Autodesk Fusion 360 part; units mm, degrees
(part 3 of 4)
sketch "Skizze42" plane through (0, 47, 0) normal (0, 1, 0) x (-1, 0, 0)
  line L0 (22.3, -10.5) -> (30, -10.5)
  line L1 (30, -10.5) -> (30, -18.5)
  line L2 (30, -18.5) -> (22.3, -18.5)
  line L3 (22.3, -18.5) -> (22.3, -10.5)
  line L4 (-37.3325, -7.5) -> (-48.5, -7.5)
  arc A0 (-48.5, -4.5) -> (-48.5, -7.5) centre (-48.5, -6) ccw
  line L5 (-48.5, -4.5) -> (-37.3325, -4.5)
  arc A1 (-37.3325, -7.5) -> (-37.3325, -4.5) centre (-37.3325, -6) ccw
  line L6 (-12.5, -6.3514) -> (-20.5, -6.3514)
  arc A2 (-20.5, -4.3514) -> (-20.5, -6.3514) centre (-20.5, -5.3514) ccw
  line L7 (-20.5, -4.3514) -> (-12.5, -4.3514)
  arc A3 (-12.5, -6.3514) -> (-12.5, -4.3514) centre (-12.5, -5.3514) ccw
  line L8 (-12.5, -24.0657) -> (-20.5, -24.0657)
  arc A4 (-20.5, -22.0657) -> (-20.5, -24.0657) centre (-20.5, -23.0657) ccw
  line L9 (-20.5, -22.0657) -> (-12.5, -22.0657)
  arc A5 (-12.5, -24.0657) -> (-12.5, -22.0657) centre (-12.5, -23.0657) ccw
  arc A6 (34, -4.5) -> (34, -7.5) centre (34, -6) ccw
  line L10 (34, -4.5) -> (45, -4.5)
  arc A7 (45, -7.5) -> (45, -4.5) centre (45, -6) ccw
  line L11 (45, -7.5) -> (34, -7.5)
  line L12 (34, 1.5) -> (45, 1.5)
  arc A8 (45, -1.5) -> (45, 1.5) centre (45, 0) ccw
  line L13 (45, -1.5) -> (34, -1.5)
  arc A9 (34, 1.5) -> (34, -1.5) centre (34, 0) ccw
  line L14 (-12.5, -19.6371) -> (-20.5, -19.6371)
  arc A10 (-20.5, -17.6371) -> (-20.5, -19.6371) centre (-20.5, -18.6371) ccw
  line L15 (-20.5, -17.6371) -> (-12.5, -17.6371)
  arc A11 (-12.5, -19.6371) -> (-12.5, -17.6371) centre (-12.5, -18.6371) ccw
  arc A12 (-20.8852, 0) -> (-20.5, -1.9228) centre (-20.5, -0.9228) ccw
  line L16 (-20.8852, 0) -> (-12.1148, 0)
  arc A13 (-12.5, -1.9228) -> (-12.1148, 0) centre (-12.5, -0.9228) ccw
  line L17 (-12.5, -1.9228) -> (-20.5, -1.9228)
  line L18 (-37.3325, -1.5) -> (-48.5, -1.5)
  arc A14 (-48.5, 1.5) -> (-48.5, -1.5) centre (-48.5, 0) ccw
  line L19 (-48.5, 1.5) -> (-37.3325, 1.5)
  arc A15 (-37.3325, -1.5) -> (-37.3325, 1.5) centre (-37.3325, 0) ccw
  line L20 (-20.5, 8.9343) -> (-12.5, 8.9343)
  arc A16 (-12.5, 6.9343) -> (-12.5, 8.9343) centre (-12.5, 7.9343) ccw
  line L21 (-12.5, 6.9343) -> (-20.5, 6.9343)
  arc A17 (-20.5, 8.9343) -> (-20.5, 6.9343) centre (-20.5, 7.9343) ccw
  line L22 (-12.5, -10.78) -> (-20.5, -10.78)
  arc A18 (-20.5, -8.78) -> (-20.5, -10.78) centre (-20.5, -9.78) ccw
  line L23 (-20.5, -8.78) -> (-12.5, -8.78)
  arc A19 (-12.5, -10.78) -> (-12.5, -8.78) centre (-12.5, -9.78) ccw
  arc A20 (34, 13.5) -> (34, 10.5) centre (34, 12) ccw
  line L24 (34, 13.5) -> (45, 13.5)
  arc A21 (45, 10.5) -> (45, 13.5) centre (45, 12) ccw
  line L25 (45, 10.5) -> (34, 10.5)
  arc A22 (34, -10.5) -> (34, -13.5) centre (34, -12) ccw
  line L26 (34, -10.5) -> (45, -10.5)
  arc A23 (45, -13.5) -> (45, -10.5) centre (45, -12) ccw
  line L27 (45, -13.5) -> (34, -13.5)
  arc A24 (34, 7.5) -> (34, 4.5) centre (34, 6) ccw
  line L28 (34, 7.5) -> (45, 7.5)
  arc A25 (45, 4.5) -> (45, 7.5) centre (45, 6) ccw
  line L29 (45, 4.5) -> (34, 4.5)
  line L30 (-12.5, -15.2086) -> (-20.5, -15.2086)
  arc A26 (-20.5, -13.2086) -> (-20.5, -15.2086) centre (-20.5, -14.2086) ccw
  line L31 (-20.5, -13.2086) -> (-12.5, -13.2086)
  arc A27 (-12.5, -15.2086) -> (-12.5, -13.2086) centre (-12.5, -14.2086) ccw
  line L32 (-12.5, 2.5057) -> (-20.5, 2.5057)
  arc A28 (-20.5, 4.5057) -> (-20.5, 2.5057) centre (-20.5, 3.5057) ccw
  line L33 (-20.5, 4.5057) -> (-12.5, 4.5057)
  arc A29 (-12.5, 2.5057) -> (-12.5, 4.5057) centre (-12.5, 3.5057) ccw
  line L34 (-37.3325, 4.5) -> (-48.5, 4.5)
  arc A30 (-48.5, 7.5) -> (-48.5, 4.5) centre (-48.5, 6) ccw
  line L35 (-48.5, 7.5) -> (-37.3325, 7.5)
  arc A31 (-37.3325, 4.5) -> (-37.3325, 7.5) centre (-37.3325, 6) ccw
  line L36 (21.5, -1.5) -> (21.5, -23.5)
  line L37 (21.5, -23.5) -> (-5.5, -23.5)
  line L38 (-5.5, -23.5) -> (-5.5, -1.5)
  line L39 (-5.5, -1.5) -> (21.5, -1.5)
  circle A32 centre (-36, 14.5) radius 1.9
  circle A33 centre (36, 25) radius 1.9
  circle A34 centre (36, -25) radius 1.9
  circle A35 centre (-36, -14.5) radius 1.9
  line L40 (-12, 21.5) -> (-12, 11.5)
  line L41 (-12, 11.5) -> (-21, 11.5)
  line L42 (-21, 11.5) -> (-21, 21.5)
  line L43 (-21, 21.5) -> (-22.5, 21.5)
  line L44 (-22.5, 21.5) -> (-22.5, 27.5)
  line L45 (-22.5, 27.5) -> (-32.5, 27.5)
  line L46 (-32.5, 27.5) -> (-32.5, 19)
  arc A36 (-33.5, 18) -> (-32.5, 19) centre (-33.5, 19) ccw
  line L47 (-33.5, 18) -> (-40.5, 18)
  line L48 (-40.5, 18) -> (-40.5, 11)
  line L49 (-40.5, 11) -> (-56.5, 11)
  line L50 (-56.5, 11) -> (-56.5, -11)
  line L51 (-56.5, -11) -> (-40.5, -11)
  line L52 (-40.5, -11) -> (-40.5, -18)
  line L53 (-40.5, -18) -> (-33.5, -18)
  arc A37 (-32.5, -19) -> (-33.5, -18) centre (-33.5, -19) ccw
  line L54 (-32.5, -19) -> (-32.5, -27.5)
  line L55 (-32.5, -27.5) -> (32.5, -27.5)
  line L56 (32.5, -27.5) -> (33.8276, -28.3587)
  arc A38 (33.8276, -28.3587) -> (39.5022, -26.9326) centre (36, -25) ccw
  line L57 (39.5022, -26.9326) -> (42.5, -21.5)
  line L58 (42.5, -21.5) -> (57.5, -6.5)
  line L59 (57.5, -6.5) -> (57.5, 6.5)
  line L60 (57.5, 6.5) -> (42.5, 21.5)
  line L61 (42.5, 21.5) -> (39.5022, 26.9326)
  arc A39 (39.5022, 26.9326) -> (33.8276, 28.3587) centre (36, 25) ccw
  line L62 (33.8276, 28.3587) -> (32.5, 27.5)
  line L63 (32.5, 27.5) -> (-10.5, 27.5)
  line L64 (-10.5, 27.5) -> (-10.5, 21.5)
  line L65 (-10.5, 21.5) -> (-12, 21.5)
  circle A40 centre (3.5, 16) radius 6.5
  line L66 (51.5218, -5) -> (57.5, -5)
  line L67 (57.5, -5) -> (57.5, -6.5)
  line L68 (57.5, -6.5) -> (42.5, -21.5)
  line L69 (32.5, -27.5) -> (-32.5, -27.5)
  line L70 (-32.5, -27.5) -> (-32.5, -19)
  line L71 (-32.5, -19) -> (-31, -19)
  line L72 (-31, -19) -> (-31, -26)
  line L73 (-31, -26) -> (-23, -26)
  line L74 (-23, -26) -> (23, -26)
  line L75 (23, -26) -> (31, -26)
  line L76 (31, -26) -> (31, -20)
  line L77 (31, -20) -> (41.8787, -20)
  line L78 (41.8787, -20) -> (51.5218, -10.3569)
  line L79 (51.5218, -10.3569) -> (51.5218, -5)
  circle A41 centre (36, -25) radius 1.9
  line L80 (57.5, 5) -> (51.5218, 5)
  line L81 (51.5218, 5) -> (51.5218, 10.3569)
  line L82 (51.5218, 10.3569) -> (41.8787, 20)
  line L83 (41.8787, 20) -> (31, 20)
  line L84 (31, 20) -> (31, 26)
  line L85 (31, 26) -> (-31, 26)
  line L86 (-31, 26) -> (-31, 19)
  line L87 (-31, 19) -> (-32.5, 19)
  line L88 (-32.5, 19) -> (-32.5, 27.5)
  line L89 (-32.5, 27.5) -> (32.5, 27.5)
  line L90 (42.5, 21.5) -> (57.5, 6.5)
  line L91 (57.5, 6.5) -> (57.5, 5)
  circle A42 centre (36, 25) radius 1.9
  line L92 (-51.5, 5) -> (-56.5, 5)
  line L93 (-56.5, 5) -> (-56.5, 11)
  line L94 (-56.5, 11) -> (-40.5, 11)
  line L95 (-38.5, 18) -> (-33.5, 18)
  arc A43 (-33.5, 18) -> (-32.5, 19) centre (-33.5, 19) ccw
  line L96 (-32.5, 19) -> (-31, 19)
  line L97 (-31, 19) -> (-31, 9.5)
  line L98 (-31, 9.5) -> (-51.5, 9.5)
  line L99 (-51.5, 9.5) -> (-51.5, 5)
  circle A44 centre (-36, 14.5) radius 1.9
  line L100 (-56.5, -5) -> (-51.5, -5)
  line L101 (-51.5, -5) -> (-51.5, -9.5)
  line L102 (-51.5, -9.5) -> (-31, -9.5)
  line L103 (-31, -9.5) -> (-31, -19)
  line L104 (-31, -19) -> (-32.5, -19)
  arc A45 (-32.5, -19) -> (-33.5, -18) centre (-33.5, -19) ccw
  line L105 (-33.5, -18) -> (-38.5, -18)
  line L106 (-40.5, -11) -> (-56.5, -11)
  line L107 (-56.5, -11) -> (-56.5, -5)
  circle A46 centre (-36, -14.5) radius 1.9
  circle A47 centre (36, 25) radius 4
  circle A48 centre (-36, 14.5) radius 3.5
  circle A49 centre (-36, -14.5) radius 3.5
  line L108 (-32.5, 19) -> (-32.5, 14.5)
  line L109 (-40.5, 11) -> (-36, 11)
  line L110 (-40.5, -11) -> (-36, -11)
  line L111 (-32.5, -19) -> (-32.5, -14.5)
  line L112 (32, 25) -> (32, 27.5)
  line L113 (36, 21) -> (43, 21)
  line L114 (-1.75, 0) -> (-22.5, 0)
  line L115 (36, -21) -> (43, -21)
  circle A50 centre (36, -25) radius 4
  line L116 (32, -25) -> (32, -27.5)
  line L117 (42.5, -21.5) -> (38.922, -26.9266)
  arc A51 (34.8649, -28.3108) -> (38.922, -26.9266) centre (36, -25) ccw
  line L118 (34.8649, -28.3108) -> (32.5, -27.5)
  line L119 (32.5, 27.5) -> (34.8649, 28.3108)
  arc A52 (38.922, 26.9266) -> (34.8649, 28.3108) centre (36, 25) ccw
  line L120 (38.922, 26.9266) -> (42.5, 21.5)
  arc A53 (-40.5, 11) -> (-39.5, 12) centre (-40.5, 12) ccw
  line L121 (-39.5, 12) -> (-39.5, 17)
  arc A54 (-38.5, 18) -> (-39.5, 17) centre (-38.5, 17) ccw
  arc A55 (-39.5, -17) -> (-38.5, -18) centre (-38.5, -17) ccw
  line L122 (-39.5, -17) -> (-39.5, -12)
  arc A56 (-39.5, -12) -> (-40.5, -11) centre (-40.5, -12) ccw
  dimension "d212" = 7
  dimension "d213" = 7
  measures "d212" diameter of A48
  measures "d213" diameter of A49
extrude "Extrusion42" cut sketch "Skizze42" against normal blind 13.5 contours L63 L89 A47 L112 L119 | L62 A47 L119 | A47 L119 A52 L120 | A39 A47 L119 A52 L120 | L60 L90 A47 L113 L120 | A36 L47 L95 A43 A48 L108 | L61 A47 L120 | A48 | L47 L95 A48 L121 A54 | A48 L109 A53 L121 | L47 L48 A53 L121 A54 | L58 L68 L115 A50 L117 | L57 A50 L117 | A50 L117 A51 L118 | L52 L53 A55 L122 A56 | A49 L110 L122 A56 | A38 A50 L117 A51 L118 | L55 L69 A50 L116 L118 | A49 | L56 A50 L118 | L53 L105 A49 A55 L122 | L53 A37 A45 L105 A49 L111 bodies 2
fillet "Abrundung2" radius 1 8 edges at (40.5, 10.75, 18) (40.5, 10.75, 11) (40.5, 10.75, -11) (40.5, 10.75, -18) (40.5, 29, 18) (40.5, 29, 11) (40.5, 29, -11) (40.5, 29, -18) on bodies 1 2
sketch "Skizze43" plane through (-32, 0, 32) normal (-0.707107, 0, 0.707107) x (0.707107, 0, 0.707107)
  line L0 (-15.5563, 33.5) -> (-15.5563, 47)
  line L1 (-15.5563, 47) -> (-36.0624, 47)
  line L2 (-36.0624, 47) -> (-36.0624, 16)
  line L3 (-36.0624, 16) -> (-14.8492, 16)
  line L4 (-14.8492, 19) -> (-14.8492, 33.5)
  line L5 (-14.8492, 33.5) -> (-15.5563, 33.5)
  circle A0 centre (-21.4706, 18) radius 2
  line L6 (-29.108, 16) -> (-29.108, 45)
  line L7 (-29.108, 45) -> (-15.4706, 45)
  line L8 (-15.4706, 45) -> (-15.4706, 16)
  line L9 (-15.4706, 16) -> (-29.108, 16)
  line L10 (-14.8492, 16) -> (-36.0624, 16)
  line L11 (-23.0518, 16) -> (-20.1969, 16)
  line L12 (-23.4706, 16) -> (-19.4706, 16)
  line L13 (-19.4706, 16) -> (-19.4706, 18)
  line L14 (-19.4706, 18) -> (-23.4706, 18)
  line L15 (-23.4706, 18) -> (-23.4706, 16)
  line L16 (-14.8492, 16) -> (-14.8492, 19)
  dimension "d217" = 4
  dimension "d223" = 6
  measures "d217" diameter of A0
  measures "d223" distance of L8
extrude "Extrusion43" cut sketch "Skizze43" against normal blind 2 contours L3 A0 L9 L10 L11 L12 L13 | L3 A0 L9 L10 L11 L12 L15 | A0 L14 | A0 L14 bodies 2
sketch "Sketch44" plane through (0, 47, 0) normal (0, 1, 0) x (-1, 0, 0)
  circle A0 centre (3.5, 16) radius 6.5
  line L0 (21.5, -1.5) -> (21.5, -23.5)
  line L1 (21.5, -23.5) -> (-5.5, -23.5)
  line L2 (-5.5, -23.5) -> (-5.5, -1.5)
  line L3 (-5.5, -1.5) -> (21.5, -1.5)
  line L4 (-37.3325, 4.5) -> (-48.5, 4.5)
  arc A1 (-48.5, 7.5) -> (-48.5, 4.5) centre (-48.5, 6) ccw
  line L5 (-48.5, 7.5) -> (-37.3325, 7.5)
  arc A2 (-37.3325, 4.5) -> (-37.3325, 7.5) centre (-37.3325, 6) ccw
  line L6 (-12.5, 2.5057) -> (-20.5, 2.5057)
  arc A3 (-20.5, 4.5057) -> (-20.5, 2.5057) centre (-20.5, 3.5057) ccw
  line L7 (-20.5, 4.5057) -> (-12.5, 4.5057)
  arc A4 (-12.5, 2.5057) -> (-12.5, 4.5057) centre (-12.5, 3.5057) ccw
  line L8 (-12.5, -15.2086) -> (-20.5, -15.2086)
  arc A5 (-20.5, -13.2086) -> (-20.5, -15.2086) centre (-20.5, -14.2086) ccw
  line L9 (-20.5, -13.2086) -> (-12.5, -13.2086)
  arc A6 (-12.5, -15.2086) -> (-12.5, -13.2086) centre (-12.5, -14.2086) ccw
  arc A7 (34, 7.5) -> (34, 4.5) centre (34, 6) ccw
  line L10 (34, 7.5) -> (45, 7.5)
  arc A8 (45, 4.5) -> (45, 7.5) centre (45, 6) ccw
  line L11 (45, 4.5) -> (34, 4.5)
  arc A9 (34, -10.5) -> (34, -13.5) centre (34, -12) ccw
  line L12 (34, -10.5) -> (45, -10.5)
  arc A10 (45, -13.5) -> (45, -10.5) centre (45, -12) ccw
  line L13 (45, -13.5) -> (34, -13.5)
  arc A11 (34, 13.5) -> (34, 10.5) centre (34, 12) ccw
  line L14 (34, 13.5) -> (45, 13.5)
  arc A12 (45, 10.5) -> (45, 13.5) centre (45, 12) ccw
  line L15 (45, 10.5) -> (34, 10.5)
  line L16 (-12.5, -10.78) -> (-20.5, -10.78)
  arc A13 (-20.5, -8.78) -> (-20.5, -10.78) centre (-20.5, -9.78) ccw
  line L17 (-20.5, -8.78) -> (-12.5, -8.78)
  arc A14 (-12.5, -10.78) -> (-12.5, -8.78) centre (-12.5, -9.78) ccw
  line L18 (-20.5, 8.9343) -> (-12.5, 8.9343)
  arc A15 (-12.5, 6.9343) -> (-12.5, 8.9343) centre (-12.5, 7.9343) ccw
  line L19 (-12.5, 6.9343) -> (-20.5, 6.9343)
  arc A16 (-20.5, 8.9343) -> (-20.5, 6.9343) centre (-20.5, 7.9343) ccw
  line L20 (-37.3325, -1.5) -> (-48.5, -1.5)
  arc A17 (-48.5, 1.5) -> (-48.5, -1.5) centre (-48.5, 0) ccw
  line L21 (-48.5, 1.5) -> (-37.3325, 1.5)
  arc A18 (-37.3325, -1.5) -> (-37.3325, 1.5) centre (-37.3325, 0) ccw
  arc A19 (-20.8852, 0) -> (-20.5, -1.9228) centre (-20.5, -0.9228) ccw
  line L22 (-20.8852, 0) -> (-12.1148, 0)
  arc A20 (-12.5, -1.9228) -> (-12.1148, 0) centre (-12.5, -0.9228) ccw
  line L23 (-12.5, -1.9228) -> (-20.5, -1.9228)
  line L24 (-12.5, -19.6371) -> (-20.5, -19.6371)
  arc A21 (-20.5, -17.6371) -> (-20.5, -19.6371) centre (-20.5, -18.6371) ccw
  line L25 (-20.5, -17.6371) -> (-12.5, -17.6371)
  arc A22 (-12.5, -19.6371) -> (-12.5, -17.6371) centre (-12.5, -18.6371) ccw
  line L26 (34, 1.5) -> (45, 1.5)
  arc A23 (45, -1.5) -> (45, 1.5) centre (45, 0) ccw
  line L27 (45, -1.5) -> (34, -1.5)
  arc A24 (34, 1.5) -> (34, -1.5) centre (34, 0) ccw
  arc A25 (34, -4.5) -> (34, -7.5) centre (34, -6) ccw
  line L28 (34, -4.5) -> (45, -4.5)
  arc A26 (45, -7.5) -> (45, -4.5) centre (45, -6) ccw
  line L29 (45, -7.5) -> (34, -7.5)
  line L30 (-12.5, -24.0657) -> (-20.5, -24.0657)
  arc A27 (-20.5, -22.0657) -> (-20.5, -24.0657) centre (-20.5, -23.0657) ccw
  line L31 (-20.5, -22.0657) -> (-12.5, -22.0657)
  arc A28 (-12.5, -24.0657) -> (-12.5, -22.0657) centre (-12.5, -23.0657) ccw
  line L32 (-12.5, -6.3514) -> (-20.5, -6.3514)
  arc A29 (-20.5, -4.3514) -> (-20.5, -6.3514) centre (-20.5, -5.3514) ccw
  line L33 (-20.5, -4.3514) -> (-12.5, -4.3514)
  arc A30 (-12.5, -6.3514) -> (-12.5, -4.3514) centre (-12.5, -5.3514) ccw
  line L34 (-37.3325, -7.5) -> (-48.5, -7.5)
  arc A31 (-48.5, -4.5) -> (-48.5, -7.5) centre (-48.5, -6) ccw
  line L35 (-48.5, -4.5) -> (-37.3325, -4.5)
  arc A32 (-37.3325, -7.5) -> (-37.3325, -4.5) centre (-37.3325, -6) ccw
  line L36 (22.3, -10.5) -> (30, -10.5)
  line L37 (30, -10.5) -> (30, -18.5)
  line L38 (30, -18.5) -> (22.3, -18.5)
  line L39 (22.3, -18.5) -> (22.3, -10.5)
  line L40 (-32.5, 27.5) -> (-32.5, 14.5)
  arc A33 (-36, 11) -> (-32.5, 14.5) centre (-36, 14.5) ccw
  line L41 (-36, 11) -> (-56.5, 11)
  line L42 (-56.5, 11) -> (-56.5, -11)
  line L43 (-56.5, -11) -> (-36, -11)
  arc A34 (-32.5, -14.5) -> (-36, -11) centre (-36, -14.5) ccw
  line L44 (-32.5, -14.5) -> (-32.5, -27.5)
  line L45 (-32.5, -27.5) -> (32, -27.5)
  line L46 (32, -27.5) -> (32, -25)
  arc A35 (36, -21) -> (32, -25) centre (36, -25) ccw
  line L47 (36, -21) -> (43, -21)
  line L48 (43, -21) -> (57.5, -6.5)
  line L49 (57.5, -6.5) -> (57.5, 6.5)
  line L50 (57.5, 6.5) -> (43, 21)
  line L51 (43, 21) -> (36, 21)
  arc A36 (32, 25) -> (36, 21) centre (36, 25) ccw
  line L52 (32, 25) -> (32, 27.5)
  line L53 (32, 27.5) -> (-10.5, 27.5)
  line L54 (-10.5, 27.5) -> (-10.5, 21.5)
  line L55 (-10.5, 21.5) -> (-12, 21.5)
  line L56 (-12, 21.5) -> (-12, 11.5)
  line L57 (-12, 11.5) -> (-21, 11.5)
  line L58 (-21, 11.5) -> (-21, 21.5)
  line L59 (-21, 21.5) -> (-22.5, 21.5)
  line L60 (-22.5, 21.5) -> (-22.5, 27.5)
  line L61 (-22.5, 27.5) -> (-32.5, 27.5)
  line L62 (-12.5, -4.3514) -> (-20.5, -4.3514)
  line L63 (-20.5, -4.3514) -> (-20.5, -7.58)
  line L64 (-20.5, -7.58) -> (-12.5, -7.58)
  line L65 (-12.5, -7.58) -> (-12.5, -4.3514)
  dimension "d220" = 1.2
  measures "d220" distance of L17 L64
extrude "Extrude44" cut sketch "Sketch44" against normal blind 2 contours L32 L63 L64 L65 bodies 2
sketch "Skizze46" plane through (0, 0, -27.5) normal (0, 0, -1) x (-1, 0, 0)
  line L0 (-32.5, 0) -> (32.5, 0)
  line L1 (32.5, 0) -> (32.5, 16)
  line L2 (32.5, 16) -> (-32.5, 16)
  line L3 (-32.5, 16) -> (-32.5, 0)
  line L4 (-20, 2) -> (20, 2)
  line L5 (20, 2) -> (20, 42)
  line L6 (20, 42) -> (-20, 42)
  line L7 (-20, 42) -> (-20, 2)
  circle A0 centre (0, 22) radius 19
  circle A1 centre (-16, 38) radius 1.75
  circle A2 centre (-16, 6) radius 1.75
  line L8 (0, 1.75) -> (0, 22.5)
  circle A3 centre (16, 38) radius 1.75
  circle A4 centre (16, 6) radius 1.75
  circle A5 centre (0, 22) radius 2
  line L9 (0, 22) -> (-16, 6)
  line L10 (-16, 6) -> (-16.7071, 6.7071)
  line L11 (-16.7071, 6.7071) -> (-0.7071, 22.7071)
  line L12 (-0.7071, 22.7071) -> (0, 22)
  line L13 (0, 22) -> (-16, 6)
  line L14 (-16, 6) -> (-15.2929, 5.2929)
  line L15 (-15.2929, 5.2929) -> (0.7071, 21.2929)
  line L16 (0.7071, 21.2929) -> (0, 22)
  line L17 (15.2929, 5.2929) -> (-0.7071, 21.2929)
  line L18 (16.7071, 6.7071) -> (0.7071, 22.7071)
  line L19 (16.7071, 37.2929) -> (0.7071, 21.2929)
  line L20 (15.2929, 38.7071) -> (-0.7071, 22.7071)
  line L21 (-15.2929, 38.7071) -> (0.7071, 22.7071)
  line L22 (-16.7071, 37.2929) -> (-0.7071, 21.2929)
  dimension "d224" = 40
  dimension "d225" = 40
  dimension "d226" = 12.5
  dimension "d227" = 38
  dimension "d228" = 3.5
  dimension "d229" = 20
  dimension "d230" = 20
  dimension "d231" = 4
  dimension "d232" = 4
  dimension "d233" = 3.5
  dimension "d234" = 4
  dimension "d235" = 4
  dimension "d236" = 4
  dimension "d237" = 1
  dimension "d238" = 1
  dimension "d240" = 360
  dimension "d241" = 2
  measures "d225" distance of origin
  measures "d226" distance of L3 L7
  measures "d227" diameter of A0
  measures "d228" diameter of A1
  measures "d229" distance of L7 origin
  measures "d230" distance of L4 origin
  measures "d232" distance of L7
  measures "d233" diameter of A2
  measures "d234" distance of L4
  measures "d235" distance of L7
  measures "d236" diameter of A5
  measures "d241" distance of L0 L4
extrude "Extrusion45" cut sketch "Skizze46" against normal blind 2 contours L2 A0 A5 L11 L22 | L2 A0 L11 | L2 A0 L18 | L2 A0 A5 L18 L19 | A0 A5 L20 L21 | A1 | A2 L10 L11 L14 L15 | A2 L9 L10 L11 L13 | L2 A0 L8 L17 | L2 A0 L8 L15 | L2 L8 A5 L17 | L2 L8 A5 L15 | A2 L9 L13 L14 L15 | A3 bodies 1 2
sketch "Skizze53" plane through (0, 0, -27.5) normal (0, 0, -1) x (-1, 0, 0)
  line L0 (4.5858, 16) -> (12.7093, 7.8765)
  arc A0 (-12.7093, 7.8765) -> (12.7093, 7.8765) centre (0, 22) ccw
  line L1 (-12.7093, 7.8765) -> (-4.5858, 16)
  line L2 (-4.5858, 16) -> (-7.4142, 16)
  line L3 (-7.4142, 16) -> (-14.1235, 9.2907)
  arc A1 (-18.0278, 16) -> (-14.1235, 9.2907) centre (0, 22) ccw
  line L4 (-18.0278, 16) -> (-32.5, 16)
  line L5 (-32.5, 16) -> (-32.5, 0)
  line L6 (-32.5, 0) -> (32.5, 0)
  line L7 (32.5, 0) -> (32.5, 16)
  line L8 (32.5, 16) -> (18.0278, 16)
  arc A2 (14.1235, 9.2907) -> (18.0278, 16) centre (0, 22) ccw
  line L9 (14.1235, 9.2907) -> (7.4142, 16)
  line L10 (7.4142, 16) -> (4.5858, 16)
  circle A3 centre (-16, 6) radius 1.75
  line L11 (-20, 2) -> (20, 2)
  line L12 (20, 2) -> (20, 42)
  line L13 (20, 42) -> (-20, 42)
  line L14 (-20, 42) -> (-20, 2)
  line L15 (0.5176, 20.0681) -> (4.5858, 16)
  line L16 (4.5858, 16) -> (7.4142, 16)
  line L17 (7.4142, 16) -> (1.9319, 21.4824)
  arc A4 (1.9319, 21.4824) -> (1.9319, 22.5176) centre (0, 22) ccw
  line L18 (1.9319, 22.5176) -> (14.1235, 34.7093)
  arc A5 (18.0278, 16) -> (14.1235, 34.7093) centre (0, 22) ccw
  line L19 (32.5, 19) -> (32.5, 33.5)
  line L20 (32.5, 33.5) -> (32, 33.5)
  line L21 (32, 33.5) -> (32, 47)
  line L22 (32, 47) -> (-32.5, 47)
  line L23 (-32.5, 47) -> (-32.5, 16)
  line L24 (-32.5, 16) -> (-18.0278, 16)
  arc A6 (-14.1235, 34.7093) -> (-18.0278, 16) centre (0, 22) ccw
  line L25 (-14.1235, 34.7093) -> (-1.9319, 22.5176)
  arc A7 (-1.9319, 22.5176) -> (-1.9319, 21.4824) centre (0, 22) ccw
  line L26 (-1.9319, 21.4824) -> (-7.4142, 16)
  line L27 (-7.4142, 16) -> (-4.5858, 16)
  line L28 (-4.5858, 16) -> (-0.5176, 20.0681)
  arc A8 (-0.5176, 20.0681) -> (0.5176, 20.0681) centre (0, 22) ccw
  circle A9 centre (-16, 38) radius 1.75
  circle A10 centre (16, 38) radius 1.75
  arc A11 (12.7093, 36.1235) -> (-12.7093, 36.1235) centre (0, 22) ccw
  line L29 (12.7093, 36.1235) -> (0.5176, 23.9319)
  arc A12 (0.5176, 23.9319) -> (-0.5176, 23.9319) centre (0, 22) ccw
  line L30 (-0.5176, 23.9319) -> (-12.7093, 36.1235)
  line L31 (-20, 42) -> (-13, 42)
  line L32 (-13, 42) -> (-13, 44)
  line L33 (-13, 44) -> (-20, 44)
  line L34 (-20, 44) -> (-20, 42)
  line L35 (-20, 44) -> (-22, 44)
  line L36 (-22, 44) -> (-22, 35.2606)
  line L37 (-22, 35.2606) -> (-20, 35.2606)
  line L38 (-20, 35.2606) -> (-20, 44)
  line L39 (20, 42) -> (13, 42)
  line L40 (13, 42) -> (13, 44)
  line L41 (13, 44) -> (20, 44)
  line L42 (20, 44) -> (20, 42)
  line L43 (20, 44) -> (22, 44)
  line L44 (22, 44) -> (22, 35)
  line L45 (22, 35) -> (20, 35)
  line L46 (20, 35) -> (20, 44)
  line L47 (-20, 2) -> (-13, 2)
  line L48 (-13, 2) -> (-13, 0)
  line L49 (-13, 0) -> (-20, 0)
  line L50 (-20, 0) -> (-20, 2)
  line L51 (-20, 0) -> (-22, 0)
  line L52 (-22, 0) -> (-22, 9)
  line L53 (-22, 9) -> (-20, 9)
  line L54 (-20, 9) -> (-20, 0)
  line L55 (20, 2) -> (13, 2)
  line L56 (13, 2) -> (13, 0)
  line L57 (13, 0) -> (20, 0)
  line L58 (20, 0) -> (20, 2)
  line L59 (20, 0) -> (22, 0)
  line L60 (22, 0) -> (22, 9)
  line L61 (22, 9) -> (20, 9)
  line L62 (20, 9) -> (20, 0)
  line L63 (18.0278, 16) -> (32.5, 16)
  line L64 (32.5, 16) -> (32.5, 19)
  dimension "d269" = 40
  dimension "d270" = 40
  dimension "d271" = 12.5
  dimension "d272" = 2
  dimension "d273" = 7
  dimension "d274" = 8.7394
  dimension "d275" = 2
  dimension "d276" = 7
  dimension "d277" = 9
  dimension "d278" = 2
  dimension "d279" = 7
  dimension "d280" = 2
  dimension "d281" = 9
  dimension "d282" = 7
  dimension "d283" = 9
  dimension "d284" = 2
  measures "d269" distance of origin
  measures "d271" distance of L5 L14
  measures "d272" distance of L6 L11
  measures "d273" distance of origin
  measures "d276" distance of origin
  measures "d281" distance of origin
  measures "d283" distance of origin
extrude "Extrusion54" add sketch "Skizze53" along normal blind 10.6 contours L6 L12 L58 L59 L60 L61 L62 | L12 L42 L43 L44 L45 L46 | L6 L11 L55 L56 L57 L58 L62 | L13 L39 L40 L41 L42 L46 | L14 L34 L35 L36 L37 L38 | L6 L14 L50 L51 L52 L53 L54 | L6 L11 L47 L48 L49 L50 L54 | L13 L31 L32 L33 L34 L38 bodies 1 2
sketch "Skizze54" plane through (0, 0, -38.1) normal (0, 0, -1) x (-1, 0, 0)
  line L0 (-20, 35.2606) -> (-20, 42)
  line L1 (-20, 42) -> (-13, 42)
  line L2 (-13, 42) -> (-13, 44)
  line L3 (-13, 44) -> (-22, 44)
  line L4 (-22, 44) -> (-22, 35.2606)
  line L5 (-22, 35.2606) -> (-20, 35.2606)
  line L6 (-13, 42) -> (-20, 35.2606)
  line L7 (20, 35) -> (22, 35)
  line L8 (22, 35) -> (22, 44)
  line L9 (22, 44) -> (13, 44)
  line L10 (13, 44) -> (13, 42)
  line L11 (13, 42) -> (20, 42)
  line L12 (20, 42) -> (20, 35)
  line L13 (20, 9) -> (20, 2)
  line L14 (20, 2) -> (13, 2)
  line L15 (13, 2) -> (13, 0)
  line L16 (13, 0) -> (22, 0)
  line L17 (22, 0) -> (22, 9)
  line L18 (22, 9) -> (20, 9)
  line L19 (-20, 9) -> (-22, 9)
  line L20 (-22, 9) -> (-22, 0)
  line L21 (-22, 0) -> (-13, 0)
  line L22 (-13, 0) -> (-13, 2)
  line L23 (-13, 2) -> (-20, 2)
  line L24 (-20, 2) -> (-20, 9)
  line L25 (-13, 2) -> (-20, 9)
  line L26 (13, 2) -> (20, 9)
  line L27 (13, 42) -> (20, 35)
extrude "Extrusion55" add sketch "Skizze54" along normal blind 1.5 bodies 1 2
extrude "Extrusion56" cut 1 faces at (20, 6.6667, -34.5667) along direction (1, 0, 0) blind 0.1 on bodies 1 bodies 1
extrude "Extrusion57" cut 2 faces at (-20, 37.3333, -31.0333) (-20, 4.3333, -34.5667) along direction (-1, 0, 0) blind 0.1 on bodies 1 2 bodies 1 2
extrude "Extrusion58" cut 1 faces at (31.5, 17.8333, -19) along direction (0, 0, -1) blind 0.2 on bodies 2 bodies 2
extrude "Extrusion59" cut 1 faces at (31.5, 17.8333, 19) along direction (0, 0, 1) blind 0.2 on bodies 2 bodies 2
sketch "Skizze55" plane through (0, 0, 0) normal (0, 1, 0) x (1, 0, 0)
  circle A0 centre (0, -55) radius 8
  circle A1 centre (0, -55) radius 3.15
  dimension "d297" = 16
  dimension "d298" = 6.3
  measures "d297" diameter of A0
  measures "d298" diameter of A1
extrude "Extrusion60" add sketch "Skizze55" along normal blind 4.5 separate body contours A0 | A1 makes body 3
sketch "Skizze56" plane through (0, 4.5, 0) normal (0, 1, 0) x (-1, 0, 0)
  circle A0 centre (0, 55) radius 8
  circle A1 centre (0, 55) radius 4.5
  dimension "d301" = 9
  measures "d301" diameter of A1
extrude "Extrusion61" add sketch "Skizze56" along normal blind 6 contours A1 bodies 3
sketch "Skizze57" plane through (0, 10.5, 0) normal (0, 1, 0) x (-1, 0, 0)
  circle A0 centre (0, 55) radius 4.5
  circle A1 centre (0, 55) radius 3.15
  dimension "d304" = 6.3
  measures "d304" diameter of A1
extrude "Extrusion62" cut sketch "Skizze57" against normal blind 9.5 contours A1 bodies 3
sketch "Skizze58" plane through (0, 10.5, 0) normal (0, 1, 0) x (-1, 0, 0)
  circle A0 centre (0, 55) radius 3.15
  circle A1 centre (0, 55) radius 4.5
  line L0 (1.4214, 57.8111) -> (-3.15, 55)
  line L1 (1.8822, 59.8553) -> (-2.2247, 57.3299)
  dimension "d307" = 1.5
  measures "d307" distance of L0 L1
extrude "Extrusion63" add sketch "Skizze58" against normal blind 9.5 contours A0 L0 picked at (-0.4448, 57.4308) bodies 3
sketch "Skizze59" plane through (0, 4.5, 0) normal (0, 1, 0) x (-1, 0, 0)
  circle A0 centre (0, 55) radius 4.5
  circle A1 centre (0, 55) radius 8
  arc A2 (7.9699, 54.3066) -> (8, 55) centre (7.9561, 54.6546) ccw
  arc A3 (7.9802, 55.5619) -> (7.9015, 56.2515) centre (7.9122, 55.9034) ccw
  arc A4 (7.7941, 56.8034) -> (7.6085, 57.4721) centre (7.6734, 57.13) ccw
  arc A5 (7.416, 58.0005) -> (7.1281, 58.6319) centre (7.2458, 58.3042) ccw
  arc A6 (6.8553, 59.1236) -> (6.4721, 59.7023) centre (6.6397, 59.397) ccw
  arc A7 (6.1259, 60.1453) -> (5.6569, 60.6569) centre (5.8701, 60.3816) ccw
  arc A8 (5.2455, 61.0402) -> (4.7023, 61.4721) centre (4.9559, 61.2336) ccw
  arc A9 (4.236, 61.7864) -> (3.6319, 62.1281) centre (3.9198, 61.9321) ccw
  arc A10 (3.1223, 62.3656) -> (2.4721, 62.6085) centre (2.7871, 62.46) ccw
  arc A11 (1.9316, 62.7633) -> (1.2515, 62.9015) centre (1.5858, 62.8041) ccw
  arc A12 (0.6934, 62.9699) -> (0, 63) centre (0.3454, 62.9561) ccw
  arc A13 (-0.5619, 62.9802) -> (-1.2515, 62.9015) centre (-0.9034, 62.9122) ccw
  arc A14 (-1.8034, 62.7941) -> (-2.4721, 62.6085) centre (-2.13, 62.6734) ccw
  arc A15 (-3.0005, 62.416) -> (-3.6319, 62.1281) centre (-3.3042, 62.2458) ccw
  arc A16 (-4.1236, 61.8553) -> (-4.7023, 61.4721) centre (-4.397, 61.6397) ccw
  arc A17 (-5.1453, 61.1259) -> (-5.6569, 60.6569) centre (-5.3816, 60.8701) ccw
  arc A18 (-6.0402, 60.2455) -> (-6.4721, 59.7023) centre (-6.2336, 59.9559) ccw
  arc A19 (-6.7864, 59.236) -> (-7.1281, 58.6319) centre (-6.9321, 58.9198) ccw
  arc A20 (-7.3656, 58.1223) -> (-7.6085, 57.4721) centre (-7.46, 57.7871) ccw
  arc A21 (-7.7633, 56.9316) -> (-7.9015, 56.2515) centre (-7.8041, 56.5858) ccw
  arc A22 (-7.9699, 55.6934) -> (-8, 55) centre (-7.9561, 55.3454) ccw
  arc A23 (-7.9802, 54.4381) -> (-7.9015, 53.7485) centre (-7.9122, 54.0966) ccw
  arc A24 (-7.7941, 53.1966) -> (-7.6085, 52.5279) centre (-7.6734, 52.87) ccw
  arc A25 (-7.416, 51.9995) -> (-7.1281, 51.3681) centre (-7.2458, 51.6958) ccw
  arc A26 (-6.8553, 50.8764) -> (-6.4721, 50.2977) centre (-6.6397, 50.603) ccw
  arc A27 (-6.1259, 49.8547) -> (-5.6569, 49.3431) centre (-5.8701, 49.6184) ccw
  arc A28 (-5.2455, 48.9598) -> (-4.7023, 48.5279) centre (-4.9559, 48.7664) ccw
  arc A29 (-4.236, 48.2136) -> (-3.6319, 47.8719) centre (-3.9198, 48.0679) ccw
  arc A30 (-3.1223, 47.6344) -> (-2.4721, 47.3915) centre (-2.7871, 47.54) ccw
  arc A31 (-1.9316, 47.2367) -> (-1.2515, 47.0985) centre (-1.5858, 47.1959) ccw
  arc A32 (-0.6934, 47.0301) -> (0, 47) centre (-0.3454, 47.0439) ccw
  arc A33 (0.5619, 47.0198) -> (1.2515, 47.0985) centre (0.9034, 47.0878) ccw
  arc A34 (1.8034, 47.2059) -> (2.4721, 47.3915) centre (2.13, 47.3266) ccw
  arc A35 (3.0005, 47.584) -> (3.6319, 47.8719) centre (3.3042, 47.7542) ccw
  arc A36 (4.1236, 48.1447) -> (4.7023, 48.5279) centre (4.397, 48.3603) ccw
  arc A37 (5.1453, 48.8741) -> (5.6569, 49.3431) centre (5.3816, 49.1299) ccw
  arc A38 (6.0402, 49.7545) -> (6.4721, 50.2977) centre (6.2336, 50.0441) ccw
  arc A39 (6.7864, 50.764) -> (7.1281, 51.3681) centre (6.9321, 51.0802) ccw
  arc A40 (7.3656, 51.8777) -> (7.6085, 52.5279) centre (7.46, 52.2129) ccw
  arc A41 (7.7633, 53.0684) -> (7.9015, 53.7485) centre (7.8041, 53.4142) ccw
  dimension "d311" = 360
extrude "Extrusion64" add sketch "Skizze59" against normal blind 4.5 contours A1 A2 | A1 A3 | A1 A41 | A1 A4 | A1 A40 | A1 A5 | A1 A39 | A1 A6 | A1 A38 | A1 A7 | A1 A37 | A1 A8 | A1 A36 | A1 A9 | A1 A35 | A1 A10 | A1 A34 | A1 A11 | A1 A33 | A1 A12 | A1 A32 | A1 A13 | A1 A31 | A1 A14 | A1 A30 | A1 A15 | A1 A29 | A1 A16 | A1 A28 | A1 A17 | A1 A27 | A1 A18 | A1 A26 | A1 A19 | A1 A25 | A1 A20 | A1 A24 | A1 A21 | A1 A23 | A1 A22 bodies 3
sketch "Skizze60" plane through (0, 0, 0) normal (0, -1, 0) x (1, 0, 0)
  arc A0 (-6.1259, 60.1453) -> (-6.4721, 59.7023) centre (0, 55) ccw
  arc A1 (-6.4721, 59.7023) -> (-6.8553, 59.1236) centre (-6.6397, 59.397) ccw
  arc A2 (-6.8553, 59.1236) -> (-7.1281, 58.6319) centre (0, 55) ccw
  arc A3 (-7.1281, 58.6319) -> (-7.416, 58.0005) centre (-7.2458, 58.3042) ccw
  arc A4 (-7.416, 58.0005) -> (-7.6085, 57.4721) centre (0, 55) ccw
  arc A5 (-7.6085, 57.4721) -> (-7.7941, 56.8034) centre (-7.6734, 57.13) ccw
  arc A6 (-7.7941, 56.8034) -> (-7.9015, 56.2515) centre (0, 55) ccw
  arc A7 (-7.9015, 56.2515) -> (-7.9802, 55.5619) centre (-7.9122, 55.9034) ccw
  arc A8 (-7.9802, 55.5619) -> (-8, 55) centre (0, 55) ccw
  arc A9 (-8, 55) -> (-7.9699, 54.3066) centre (-7.9561, 54.6546) ccw
  arc A10 (-7.9699, 54.3066) -> (-7.9015, 53.7485) centre (0, 55) ccw
  arc A11 (-7.9015, 53.7485) -> (-7.7633, 53.0684) centre (-7.8041, 53.4142) ccw
  arc A12 (-7.7633, 53.0684) -> (-7.6085, 52.5279) centre (0, 55) ccw
  arc A13 (-7.6085, 52.5279) -> (-7.3656, 51.8777) centre (-7.46, 52.2129) ccw
  arc A14 (-7.3656, 51.8777) -> (-7.1281, 51.3681) centre (0, 55) ccw
  arc A15 (-7.1281, 51.3681) -> (-6.7864, 50.764) centre (-6.9321, 51.0802) ccw
  arc A16 (-6.7864, 50.764) -> (-6.4721, 50.2977) centre (0, 55) ccw
  arc A17 (-6.4721, 50.2977) -> (-6.0402, 49.7545) centre (-6.2336, 50.0441) ccw
  arc A18 (-6.0402, 49.7545) -> (-5.6569, 49.3431) centre (0, 55) ccw
  arc A19 (-5.6569, 49.3431) -> (-5.1453, 48.8741) centre (-5.3816, 49.1299) ccw
  arc A20 (-5.1453, 48.8741) -> (-4.7023, 48.5279) centre (0, 55) ccw
  arc A21 (-4.7023, 48.5279) -> (-4.1236, 48.1447) centre (-4.397, 48.3603) ccw
  arc A22 (-4.1236, 48.1447) -> (-3.6319, 47.8719) centre (0, 55) ccw
  arc A23 (-3.6319, 47.8719) -> (-3.0005, 47.584) centre (-3.3042, 47.7542) ccw
  arc A24 (-3.0005, 47.584) -> (-2.4721, 47.3915) centre (0, 55) ccw
  arc A25 (-2.4721, 47.3915) -> (-1.8034, 47.2059) centre (-2.13, 47.3266) ccw
  arc A26 (-1.8034, 47.2059) -> (-1.2515, 47.0985) centre (0, 55) ccw
  arc A27 (-1.2515, 47.0985) -> (-0.5619, 47.0198) centre (-0.9034, 47.0878) ccw
  arc A28 (-0.5619, 47.0198) -> (0, 47) centre (0, 55) ccw
  arc A29 (0, 47) -> (0.6934, 47.0301) centre (0.3454, 47.0439) ccw
  arc A30 (0.6934, 47.0301) -> (1.2515, 47.0985) centre (0, 55) ccw
  arc A31 (1.2515, 47.0985) -> (1.9316, 47.2367) centre (1.5858, 47.1959) ccw
  arc A32 (1.9316, 47.2367) -> (2.4721, 47.3915) centre (0, 55) ccw
  arc A33 (2.4721, 47.3915) -> (3.1223, 47.6344) centre (2.7871, 47.54) ccw
  arc A34 (3.1223, 47.6344) -> (3.6319, 47.8719) centre (0, 55) ccw
  arc A35 (3.6319, 47.8719) -> (4.236, 48.2136) centre (3.9198, 48.0679) ccw
  arc A36 (4.236, 48.2136) -> (4.7023, 48.5279) centre (0, 55) ccw
  arc A37 (4.7023, 48.5279) -> (5.2455, 48.9598) centre (4.9559, 48.7664) ccw
  arc A38 (5.2455, 48.9598) -> (5.6569, 49.3431) centre (0, 55) ccw
  arc A39 (5.6569, 49.3431) -> (6.1259, 49.8547) centre (5.8701, 49.6184) ccw
  arc A40 (6.1259, 49.8547) -> (6.4721, 50.2977) centre (0, 55) ccw
  arc A41 (6.4721, 50.2977) -> (6.8553, 50.8764) centre (6.6397, 50.603) ccw
  arc A42 (6.8553, 50.8764) -> (7.1281, 51.3681) centre (0, 55) ccw
  arc A43 (7.1281, 51.3681) -> (7.416, 51.9995) centre (7.2458, 51.6958) ccw
  arc A44 (7.416, 51.9995) -> (7.6085, 52.5279) centre (0, 55) ccw
  arc A45 (7.6085, 52.5279) -> (7.7941, 53.1966) centre (7.6734, 52.87) ccw
  arc A46 (7.7941, 53.1966) -> (7.9015, 53.7485) centre (0, 55) ccw
  arc A47 (7.9015, 53.7485) -> (7.9802, 54.4381) centre (7.9122, 54.0966) ccw
  arc A48 (7.9802, 54.4381) -> (8, 55) centre (0, 55) ccw
  arc A49 (8, 55) -> (7.9699, 55.6934) centre (7.9561, 55.3454) ccw
  arc A50 (7.9699, 55.6934) -> (7.9015, 56.2515) centre (0, 55) ccw
  arc A51 (7.9015, 56.2515) -> (7.7633, 56.9316) centre (7.8041, 56.5858) ccw
  arc A52 (7.7633, 56.9316) -> (7.6085, 57.4721) centre (0, 55) ccw
  arc A53 (7.6085, 57.4721) -> (7.3656, 58.1223) centre (7.46, 57.7871) ccw
  arc A54 (7.3656, 58.1223) -> (7.1281, 58.6319) centre (0, 55) ccw
  arc A55 (7.1281, 58.6319) -> (6.7864, 59.236) centre (6.9321, 58.9198) ccw
  arc A56 (6.7864, 59.236) -> (6.4721, 59.7023) centre (0, 55) ccw
  arc A57 (6.4721, 59.7023) -> (6.0402, 60.2455) centre (6.2336, 59.9559) ccw
  arc A58 (6.0402, 60.2455) -> (5.6569, 60.6569) centre (0, 55) ccw
  arc A59 (5.6569, 60.6569) -> (5.1453, 61.1259) centre (5.3816, 60.8701) ccw
  arc A60 (5.1453, 61.1259) -> (4.7023, 61.4721) centre (0, 55) ccw
  arc A61 (4.7023, 61.4721) -> (4.1236, 61.8553) centre (4.397, 61.6397) ccw
  arc A62 (4.1236, 61.8553) -> (3.6319, 62.1281) centre (0, 55) ccw
  arc A63 (3.6319, 62.1281) -> (3.0005, 62.416) centre (3.3042, 62.2458) ccw
  arc A64 (3.0005, 62.416) -> (2.4721, 62.6085) centre (0, 55) ccw
  arc A65 (2.4721, 62.6085) -> (1.8034, 62.7941) centre (2.13, 62.6734) ccw
  arc A66 (1.8034, 62.7941) -> (1.2515, 62.9015) centre (0, 55) ccw
  arc A67 (1.2515, 62.9015) -> (0.5619, 62.9802) centre (0.9034, 62.9122) ccw
  arc A68 (0.5619, 62.9802) -> (0, 63) centre (0, 55) ccw
  arc A69 (0, 63) -> (-0.6934, 62.9699) centre (-0.3454, 62.9561) ccw
  arc A70 (-0.6934, 62.9699) -> (-1.2515, 62.9015) centre (0, 55) ccw
  arc A71 (-1.2515, 62.9015) -> (-1.9316, 62.7633) centre (-1.5858, 62.8041) ccw
  arc A72 (-1.9316, 62.7633) -> (-2.4721, 62.6085) centre (0, 55) ccw
  arc A73 (-2.4721, 62.6085) -> (-3.1223, 62.3656) centre (-2.7871, 62.46) ccw
  arc A74 (-3.1223, 62.3656) -> (-3.6319, 62.1281) centre (0, 55) ccw
  arc A75 (-3.6319, 62.1281) -> (-4.236, 61.7864) centre (-3.9198, 61.9321) ccw
  arc A76 (-4.236, 61.7864) -> (-4.7023, 61.4721) centre (0, 55) ccw
  arc A77 (-4.7023, 61.4721) -> (-5.2455, 61.0402) centre (-4.9559, 61.2336) ccw
  arc A78 (-5.2455, 61.0402) -> (-5.6569, 60.6569) centre (0, 55) ccw
  arc A79 (-5.6569, 60.6569) -> (-6.1259, 60.1453) centre (-5.8701, 60.3816) ccw
  circle A80 centre (0, 55) radius 8
extrude "Extrusion65" add sketch "Skizze60" along normal blind 1 contours A0 A2 A4 A6 A8 A10 A12 A14 A16 A18 A20 A22 A24 A26 A28 A30 A32 A34 A36 A38 A40 A42 A44 A46 A48 A50 A52 A54 A56 A58 A60 A62 A64 A66 A68 A70 A72 A74 A76 A78 A80 bodies 3
chamfer "Fase2" distance 1 angle 45 1 edges at (-7.4586, -1, 52.1071) on bodies 3
sketch "Skizze61" plane through (0, 0, 27.5) normal (0, 0, 1) x (1, 0, 0)
  line L0 (-32.5, 0) -> (32.5, 0)
  line L1 (32.5, 0) -> (32.5, 16)
  line L2 (32.5, 16) -> (-32.5, 16)
  line L3 (-32.5, 16) -> (-32.5, 0)
  line L4 (-9.4118, 6.9027) -> (-15.8397, 14.5631)
  arc A0 (-15.8397, 14.5631) -> (-18.1378, 12.6348) centre (-16.9888, 13.599) ccw
  line L5 (-18.1378, 12.6348) -> (-11.71, 4.9743)
  arc A1 (-11.71, 4.9743) -> (-9.4118, 6.9027) centre (-10.5609, 5.9385) ccw
  line L6 (-10.5609, 5.9385) -> (-16.9888, 13.599) construction
  line L7 (-9.1378, 12.6348) -> (-2.71, 4.9743)
  arc A2 (-6.8397, 14.5631) -> (-9.1378, 12.6348) centre (-7.9888, 13.599) ccw
  line L8 (-0.4118, 6.9027) -> (-6.8397, 14.5631)
  arc A3 (-2.71, 4.9743) -> (-0.4118, 6.9027) centre (-1.5609, 5.9385) ccw
  line L9 (-0.1378, 12.6348) -> (6.29, 4.9743)
  arc A4 (2.1603, 14.5631) -> (-0.1378, 12.6348) centre (1.0112, 13.599) ccw
  line L10 (8.5882, 6.9027) -> (2.1603, 14.5631)
  arc A5 (6.29, 4.9743) -> (8.5882, 6.9027) centre (7.4391, 5.9385) ccw
  line L11 (8.8622, 12.6348) -> (15.29, 4.9743)
  arc A6 (11.1603, 14.5631) -> (8.8622, 12.6348) centre (10.0112, 13.599) ccw
  line L12 (17.5882, 6.9027) -> (11.1603, 14.5631)
  arc A7 (15.29, 4.9743) -> (17.5882, 6.9027) centre (16.4391, 5.9385) ccw
  dimension "d317" = 3
  dimension "d320" = 27
  dimension "d321" = 0
  measures "d317" diameter of A0
extrude "Extrusion66" cut sketch "Skizze61" against normal blind 2 contours L4 A0 L5 A1 | L7 A2 L8 A3 | L9 A4 L10 A5 | L11 A6 L12 A7 bodies 1
extrude "Extrusion67" cut 1 faces at (0.1557, 1, 54.0798) along direction (0, -1, 0) blind 1 on bodies 3 bodies 3
sketch "Skizze62" plane through (0, 10.5, 0) normal (0, 1, 0) x (-1, 0, 0)
  arc A0 (-3.15, 55) -> (1.4214, 57.8111) centre (0, 55) ccw
  line L0 (-3.15, 55) -> (1.4214, 57.8111)
  circle A1 centre (0, 55) radius 4.5
  circle A2 centre (0, 55) radius 3.15
extrude "Extrusion68" add sketch "Skizze62" along normal blind 3 bodies 3
sketch "Skizze63" plane through (0, 47, 0) normal (0, 1, 0) x (-1, 0, 0)
  line L0 (-20.5, -7.58) -> (-20.5, -6.3514)
  arc A0 (-20.5, -4.3514) -> (-20.5, -6.3514) centre (-20.5, -5.3514) ccw
  line L1 (-20.5, -4.3514) -> (-12.5, -4.3514)
  arc A1 (-12.5, -6.3514) -> (-12.5, -4.3514) centre (-12.5, -5.3514) ccw
  line L2 (-12.5, -6.3514) -> (-12.5, -7.58)
  line L3 (-12.5, -7.58) -> (-20.5, -7.58)
  circle A2 centre (3.5, 16) radius 6.5
  line L4 (21.5, -1.5) -> (21.5, -23.5)
  line L5 (21.5, -23.5) -> (-5.5, -23.5)
  line L6 (-5.5, -23.5) -> (-5.5, -1.5)
  line L7 (-5.5, -1.5) -> (21.5, -1.5)
  line L8 (-37.3325, 4.5) -> (-48.5, 4.5)
  arc A3 (-48.5, 7.5) -> (-48.5, 4.5) centre (-48.5, 6) ccw
  line L9 (-48.5, 7.5) -> (-37.3325, 7.5)
  arc A4 (-37.3325, 4.5) -> (-37.3325, 7.5) centre (-37.3325, 6) ccw
  line L10 (-12.5, 2.5057) -> (-20.5, 2.5057)
  arc A5 (-20.5, 4.5057) -> (-20.5, 2.5057) centre (-20.5, 3.5057) ccw
  line L11 (-20.5, 4.5057) -> (-12.5, 4.5057)
  arc A6 (-12.5, 2.5057) -> (-12.5, 4.5057) centre (-12.5, 3.5057) ccw
  line L12 (-12.5, -15.2086) -> (-20.5, -15.2086)
  arc A7 (-20.5, -13.2086) -> (-20.5, -15.2086) centre (-20.5, -14.2086) ccw
  line L13 (-20.5, -13.2086) -> (-12.5, -13.2086)
  arc A8 (-12.5, -15.2086) -> (-12.5, -13.2086) centre (-12.5, -14.2086) ccw
  arc A9 (34, 7.5) -> (34, 4.5) centre (34, 6) ccw
  line L14 (34, 7.5) -> (45, 7.5)
  arc A10 (45, 4.5) -> (45, 7.5) centre (45, 6) ccw
  line L15 (45, 4.5) -> (34, 4.5)
  arc A11 (34, -10.5) -> (34, -13.5) centre (34, -12) ccw
  line L16 (34, -10.5) -> (45, -10.5)
  arc A12 (45, -13.5) -> (45, -10.5) centre (45, -12) ccw
  line L17 (45, -13.5) -> (34, -13.5)
  arc A13 (34, 13.5) -> (34, 10.5) centre (34, 12) ccw
  line L18 (34, 13.5) -> (45, 13.5)
  arc A14 (45, 10.5) -> (45, 13.5) centre (45, 12) ccw
  line L19 (45, 10.5) -> (34, 10.5)
  line L20 (-12.5, -10.78) -> (-20.5, -10.78)
  arc A15 (-20.5, -8.78) -> (-20.5, -10.78) centre (-20.5, -9.78) ccw
  line L21 (-20.5, -8.78) -> (-12.5, -8.78)
  arc A16 (-12.5, -10.78) -> (-12.5, -8.78) centre (-12.5, -9.78) ccw
  line L22 (-20.5, 8.9343) -> (-12.5, 8.9343)
  arc A17 (-12.5, 6.9343) -> (-12.5, 8.9343) centre (-12.5, 7.9343) ccw
  line L23 (-12.5, 6.9343) -> (-20.5, 6.9343)
  arc A18 (-20.5, 8.9343) -> (-20.5, 6.9343) centre (-20.5, 7.9343) ccw
  line L24 (-37.3325, -1.5) -> (-48.5, -1.5)
  arc A19 (-48.5, 1.5) -> (-48.5, -1.5) centre (-48.5, 0) ccw
  line L25 (-48.5, 1.5) -> (-37.3325, 1.5)
  arc A20 (-37.3325, -1.5) -> (-37.3325, 1.5) centre (-37.3325, 0) ccw
  arc A21 (-20.8852, 0) -> (-20.5, -1.9228) centre (-20.5, -0.9228) ccw
  line L26 (-20.8852, 0) -> (-12.1148, 0)
  arc A22 (-12.5, -1.9228) -> (-12.1148, 0) centre (-12.5, -0.9228) ccw
  line L27 (-12.5, -1.9228) -> (-20.5, -1.9228)
  line L28 (-12.5, -19.6371) -> (-20.5, -19.6371)
  arc A23 (-20.5, -17.6371) -> (-20.5, -19.6371) centre (-20.5, -18.6371) ccw
  line L29 (-20.5, -17.6371) -> (-12.5, -17.6371)
  arc A24 (-12.5, -19.6371) -> (-12.5, -17.6371) centre (-12.5, -18.6371) ccw
  line L30 (34, 1.5) -> (45, 1.5)
  arc A25 (45, -1.5) -> (45, 1.5) centre (45, 0) ccw
  line L31 (45, -1.5) -> (34, -1.5)
  arc A26 (34, 1.5) -> (34, -1.5) centre (34, 0) ccw
  arc A27 (34, -4.5) -> (34, -7.5) centre (34, -6) ccw
  line L32 (34, -4.5) -> (45, -4.5)
  arc A28 (45, -7.5) -> (45, -4.5) centre (45, -6) ccw
  line L33 (45, -7.5) -> (34, -7.5)
  line L34 (-12.5, -24.0657) -> (-20.5, -24.0657)
  arc A29 (-20.5, -22.0657) -> (-20.5, -24.0657) centre (-20.5, -23.0657) ccw
  line L35 (-20.5, -22.0657) -> (-12.5, -22.0657)
  arc A30 (-12.5, -24.0657) -> (-12.5, -22.0657) centre (-12.5, -23.0657) ccw
  line L36 (-37.3325, -7.5) -> (-48.5, -7.5)
  arc A31 (-48.5, -4.5) -> (-48.5, -7.5) centre (-48.5, -6) ccw
  line L37 (-48.5, -4.5) -> (-37.3325, -4.5)
  arc A32 (-37.3325, -7.5) -> (-37.3325, -4.5) centre (-37.3325, -6) ccw
  line L38 (22.3, -10.5) -> (30, -10.5)
  line L39 (30, -10.5) -> (30, -18.5)
  line L40 (30, -18.5) -> (22.3, -18.5)
  line L41 (22.3, -18.5) -> (22.3, -10.5)
  line L42 (-32.5, 27.5) -> (-32.5, 14.5)
  arc A33 (-36, 11) -> (-32.5, 14.5) centre (-36, 14.5) ccw
  line L43 (-36, 11) -> (-56.5, 11)
  line L44 (-56.5, 11) -> (-56.5, -11)
  line L45 (-56.5, -11) -> (-36, -11)
  arc A34 (-32.5, -14.5) -> (-36, -11) centre (-36, -14.5) ccw
  line L46 (-32.5, -14.5) -> (-32.5, -27.5)
  line L47 (-32.5, -27.5) -> (32, -27.5)
  line L48 (32, -27.5) -> (32, -25)
  arc A35 (36, -21) -> (32, -25) centre (36, -25) ccw
  line L49 (36, -21) -> (43, -21)
  line L50 (43, -21) -> (57.5, -6.5)
  line L51 (57.5, -6.5) -> (57.5, 6.5)
  line L52 (57.5, 6.5) -> (43, 21)
  line L53 (43, 21) -> (36, 21)
  arc A36 (32, 25) -> (36, 21) centre (36, 25) ccw
  line L54 (32, 25) -> (32, 27.5)
  line L55 (32, 27.5) -> (-10.5, 27.5)
  line L56 (-10.5, 27.5) -> (-10.5, 21.5)
  line L57 (-10.5, 21.5) -> (-12, 21.5)
  line L58 (-12, 21.5) -> (-12, 11.5)
  line L59 (-12, 11.5) -> (-21, 11.5)
  line L60 (-21, 11.5) -> (-21, 21.5)
  line L61 (-21, 21.5) -> (-22.5, 21.5)
  line L62 (-22.5, 21.5) -> (-22.5, 27.5)
  line L63 (-20.5, -22.0657) -> (-12.5, -22.0657)
  line L64 (-12.5, -19.6371) -> (-20.5, -19.6371)
  line L65 (-12.5, -22.0657) -> (-12.5, -19.6371)
  line L66 (-20.5, -22.0657) -> (-20.5, -19.6371)
  line L67 (-22.5, 27.5) -> (-32.5, 27.5)
extrude "Extrusion69" cut sketch "Skizze63" against normal blind 1 contours L28 L35 L63 L64 L65 L66 bodies 2
sketch "Skizze64" plane through (0, 0, -27.5) normal (0, 0, -1) x (-1, 0, 0)
  arc A0 (12.7093, 36.1235) -> (-12.7093, 36.1235) centre (0, 22) ccw
  line L0 (12.7093, 36.1235) -> (0.5176, 23.9319)
  arc A1 (0.5176, 23.9319) -> (-0.5176, 23.9319) centre (0, 22) ccw
  line L1 (-0.5176, 23.9319) -> (-12.7093, 36.1235)
  circle A2 centre (16, 38) radius 1.75
  circle A3 centre (-16, 38) radius 1.75
  line L2 (-13, 44) -> (-13, 42)
  line L3 (-13, 42) -> (-20, 42)
  line L4 (-20, 42) -> (-20, 35.2606)
  line L5 (-20, 35.2606) -> (-22, 35.2606)
  line L6 (-22, 35.2606) -> (-22, 44)
  line L7 (13, 44) -> (22, 44)
  line L8 (-32.5, 47) -> (-32.5, 16)
  line L9 (18.0278, 16) -> (32.5, 16)
  arc A4 (-14.1235, 34.7093) -> (-18.0278, 16) centre (0, 22) ccw
  line L10 (-14.1235, 34.7093) -> (-1.9319, 22.5176)
  arc A5 (-1.9319, 22.5176) -> (-1.9319, 21.4824) centre (0, 22) ccw
  line L11 (-1.9319, 21.4824) -> (-7.4142, 16)
  line L12 (-7.4142, 16) -> (-4.5858, 16)
  line L13 (-4.5858, 16) -> (-0.5176, 20.0681)
  arc A6 (-0.5176, 20.0681) -> (0.5176, 20.0681) centre (0, 22) ccw
  line L14 (0.5176, 20.0681) -> (4.5858, 16)
  line L15 (4.5858, 16) -> (7.4142, 16)
  line L16 (7.4142, 16) -> (1.9319, 21.4824)
  arc A7 (1.9319, 21.4824) -> (1.9319, 22.5176) centre (0, 22) ccw
  line L17 (1.9319, 22.5176) -> (14.1235, 34.7093)
  arc A8 (18.0278, 16) -> (14.1235, 34.7093) centre (0, 22) ccw
  line L18 (32.5, 19) -> (32.5, 33.5)
  line L19 (32.5, 33.5) -> (32, 33.5)
  line L20 (32, 33.5) -> (32, 47)
  line L21 (22, 44) -> (22, 35)
  line L22 (22, 35) -> (20.1, 35)
  line L23 (20.1, 35) -> (20.1, 42)
  line L24 (20.1, 42) -> (13, 42)
  line L25 (13, 42) -> (13, 44)
  line L26 (4.5858, 16) -> (0.5176, 20.0681)
  arc A9 (-0.5176, 20.0681) -> (0.5176, 20.0681) centre (0, 22) ccw
  line L27 (-0.5176, 20.0681) -> (-4.5858, 16)
  line L28 (-4.5858, 16) -> (-7.4142, 16)
  line L29 (-7.4142, 16) -> (-1.9319, 21.4824)
  arc A10 (-1.9319, 22.5176) -> (-1.9319, 21.4824) centre (0, 22) ccw
  line L30 (-1.9319, 22.5176) -> (-14.1235, 34.7093)
  arc A11 (-14.1235, 34.7093) -> (-18.0278, 16) centre (0, 22) ccw
  line L31 (-18.0278, 16) -> (-23, 16)
  line L32 (-23, 16) -> (-23, 45)
  line L33 (-23, 45) -> (23, 45)
  line L34 (23, 45) -> (23, 16)
  line L35 (23, 16) -> (18.0278, 16)
  arc A12 (18.0278, 16) -> (14.1235, 34.7093) centre (0, 22) ccw
  line L36 (14.1235, 34.7093) -> (1.9319, 22.5176)
  arc A13 (1.9319, 21.4824) -> (1.9319, 22.5176) centre (0, 22) ccw
  line L37 (1.9319, 21.4824) -> (7.4142, 16)
  line L38 (7.4142, 16) -> (4.5858, 16)
  arc A14 (12.7093, 36.1235) -> (-12.7093, 36.1235) centre (0, 22) ccw
  line L39 (-12.7093, 36.1235) -> (-0.5176, 23.9319)
  arc A15 (0.5176, 23.9319) -> (-0.5176, 23.9319) centre (0, 22) ccw
  line L40 (0.5176, 23.9319) -> (12.7093, 36.1235)
  circle A16 centre (16, 38) radius 1.75
  circle A17 centre (-16, 38) radius 1.75
  circle A18 centre (0, 22) radius 19
  line L41 (-22, 44) -> (-13, 44)
  line L42 (32.5, 16) -> (32.5, 19)
  line L43 (32, 47) -> (-32.5, 47)
  line L44 (-32.5, 16) -> (-18.0278, 16)
extrude "Extrusion70" cut sketch "Skizze64" against normal blind 2 contours L0 A1 L1 L10 A5 L11 L12 L13 A6 L14 L15 L16 A7 L17 L26 A9 L27 L28 L29 A10 L30 L36 A13 L37 L38 L39 A15 L40 A18 | A4 L10 A5 L11 L12 L13 A6 L14 L15 L16 A7 L17 A8 L26 A9 L27 L28 L29 A10 L30 A11 A12 L36 A13 L37 L38 A18 bodies 1 2
sketch "Skizze65" plane through (0, 0, -27.5) normal (0, 0, -1) x (-1, 0, 0)
  arc A0 (18.0278, 16) -> (-18.0278, 16) centre (0, 22) ccw
  line L0 (18.0278, 16) -> (32.5, 16)
  line L1 (32.5, 19) -> (32.5, 33.5)
  line L2 (32.5, 33.5) -> (32, 33.5)
  line L3 (32, 33.5) -> (32, 47)
  line L4 (32, 47) -> (-32.5, 47)
  line L5 (22, 44) -> (22, 35)
  line L6 (22, 35) -> (20.1, 35)
  line L7 (20.1, 35) -> (20.1, 42)
  line L8 (20.1, 42) -> (13, 42)
  line L9 (13, 42) -> (13, 44)
  line L10 (-13, 44) -> (-13, 42)
  line L11 (-13, 42) -> (-20, 42)
  line L12 (-20, 42) -> (-20, 35.2606)
  line L13 (-20, 35.2606) -> (-22, 35.2606)
  line L14 (-22, 35.2606) -> (-22, 44)
  line L15 (-32.5, 47) -> (-32.5, 16)
  line L16 (-32.5, 16) -> (-18.0278, 16)
  circle A1 centre (16, 38) radius 1.75
  circle A2 centre (-16, 38) radius 1.75
  circle A3 centre (-16, 38) radius 1.75
  circle A4 centre (16, 38) radius 1.75
  circle A5 centre (-16, 6) radius 1.75
  line L17 (32.5, 16) -> (32.5, 19)
  line L18 (13, 44) -> (22, 44)
  line L19 (-22, 44) -> (-13, 44)
extrude "Extrusion71" add sketch "Skizze65" against normal blind 1.5 contours A1 A4 | A2 A3 | A5 bodies 1 2
chamfer "Fase3" distance 0.5 angle 45 1 edges at (2.9368, 13.5, 56.1391) on bodies 3